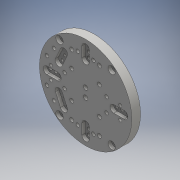
# Autodesk Inventor part: Modular Chassis
Saved by Autodesk Inventor 2016 (Build 200138000, 138)
## iProperties
Created: 2017-03-04
Part Number: Modular Chassis
Material: Generic
Document SubType Name: Modeling
Designer: Billy
Density: 1 g/cm^3
Appearance: Default
Author: Billy
Autodesk Inventor part; units mm, degrees
ref_plane "YZ Plane" through (0, 0, 0) normal (1, 0, 0) x (0, 1, 0)
ref_plane "XZ Plane" through (0, 0, 0) normal (0, 1, 0) x (-1, 0, 0)
ref_plane "XY Plane" through (0, 0, 0) normal (0, 0, 1) x (1, 0, 0)
sketch "Sketch1" plane through (0, 0, 0) normal (0, 1, 0) x (-1, 0, 0)
  circle A0 centre (15.9, 35) radius 2.25
  circle A1 centre (-15.9, 35) radius 2.25
  circle A2 centre (15.9, 16) radius 2.25
  circle A3 centre (-15.9, 16) radius 2.25
  circle A4 centre (0, 0) radius 50.3115
  circle A5 centre (15.9, -35) radius 2.25
  circle A6 centre (-15.9, -35) radius 2.25
  circle A7 centre (15.9, -16) radius 2.25
  circle A8 centre (-15.9, -16) radius 2.25
  circle A9 centre (9, 36.6994) radius 2
  circle A10 centre (-9, 36.6994) radius 2
  circle A11 centre (9, -36.6994) radius 2
  circle A12 centre (-9, -36.6994) radius 2
  circle A13 centre (39.8115, 7.366) radius 1.75
  circle A14 centre (39.8115, -7.366) radius 1.75
  circle A15 centre (-39.8115, 7.366) radius 1.75
  circle A16 centre (-39.8115, -7.366) radius 1.75
  circle A17 centre (27.8558, 21.183) radius 1.5
  circle A18 centre (30.7406, 14.8051) radius 1.5
  circle A19 centre (24.9709, 27.5609) radius 1.5
  circle A20 centre (27.8558, -21.183) radius 1.5
  circle A21 centre (30.7406, -14.8051) radius 1.5
  circle A22 centre (24.9709, -27.5609) radius 1.5
  circle A23 centre (0, 32.3115) radius 2
  circle A24 centre (0, 38.3115) radius 2
  circle A25 centre (0, 44.3115) radius 2
  circle A26 centre (-32.3115, 0) radius 2
  circle A27 centre (-38.3115, 0) radius 2
  circle A28 centre (-44.3115, 0) radius 2
  circle A29 centre (0, -32.3115) radius 2
  circle A30 centre (0, -38.3115) radius 2
  circle A31 centre (0, -44.3115) radius 2
  circle A32 centre (32.3115, 0) radius 2
  circle A33 centre (38.3115, 0) radius 2
  circle A34 centre (44.3115, 0) radius 2
  circle A35 centre (0, 5) radius 2.5
  circle A36 centre (0, -5) radius 2.5
  circle A37 centre (24.1058, 8) radius 2
  circle A38 centre (24.1058, -8) radius 2
  circle A39 centre (-24.1058, 8) radius 2
  circle A40 centre (-24.1058, -8) radius 2
  circle A41 centre (-27.8558, -21.183) radius 2
  circle A42 centre (27.886, -37.3906) radius 2
  line L0 (0, 0) -> (2.5, 0)
  circle A43 centre (27.886, 37.3906) radius 2
  circle A44 centre (44.3115, -14.732) radius 2
  circle A45 centre (44.3115, 14.732) radius 2
  line L1 (-27.8558, -21.183) -> (-36.9207, -29.0268)
  circle A46 centre (-21.8779, -28.0915) radius 2
  circle A47 centre (-33.8336, -14.2745) radius 2
  circle A48 centre (-27.9275, -33.3262) radius 2
  circle A49 centre (-33.9054, -26.4177) radius 2
  circle A50 centre (-39.8833, -19.5092) radius 2
  circle A51 centre (-27.8558, 21.183) radius 2
  circle A52 centre (-21.8779, 28.0915) radius 2
  circle A53 centre (-33.8336, 14.2745) radius 2
  circle A54 centre (-27.9275, 33.3262) radius 2
  circle A55 centre (-33.9054, 26.4177) radius 2
  circle A56 centre (-39.8833, 19.5092) radius 2
  circle A57 centre (36.0988, -26.0613) radius 2
  circle A58 centre (36.0988, 26.0613) radius 2
  point P0 (-36.9207, 29.0268)
  dimension "d47" = 360
  dimension "d64" = 8
  dimension "d69" = 4
  dimension "d70" = 4
  constraints: 59 centre point, 9 symmetric about line, 4 end point, 1 horizontal, 40 other
  measures "d64" distance of A46.centre A48.centre
  measures "d69" diameter of A57
  measures "d70" diameter of A58
extrude "Extrusion1" add sketch "Sketch1" along normal blind 10
sketch "Sketch2" plane through (0, 10, 0) normal (0, 1, 0) x (1, 0, 0)
  circle A0 centre (0, 5) radius 2.5
  circle A1 centre (0, -5) radius 2.5
  circle A2 centre (15.9, 16) radius 2.25
  circle A3 centre (-15.9, 16) radius 2.25
  circle A4 centre (15.9, 35) radius 2.25
  circle A5 centre (-15.9, 35) radius 2.25
  circle A6 centre (15.9, -16) radius 2.25
  circle A7 centre (-15.9, -16) radius 2.25
  circle A8 centre (15.9, -35) radius 2.25
  circle A9 centre (-36.0988, -26.0613) radius 2
  circle A10 centre (-36.0988, 26.0613) radius 2
  circle A11 centre (27.9275, -33.3262) radius 2
  circle A12 centre (39.8833, -19.5092) radius 2
  circle A13 centre (33.8336, -14.2745) radius 2
  circle A14 centre (27.8558, -21.183) radius 2
  circle A15 centre (33.9054, -26.4177) radius 2
  circle A16 centre (21.8779, -28.0915) radius 2
  circle A17 centre (39.8833, 19.5092) radius 2
  circle A18 centre (33.9054, 26.4177) radius 2
  circle A19 centre (27.9275, 33.3262) radius 2
  circle A20 centre (33.8336, 14.2745) radius 2
  circle A21 centre (21.8779, 28.0915) radius 2
  circle A22 centre (-44.3115, -14.732) radius 2
  circle A23 centre (-44.3115, 14.732) radius 2
  circle A24 centre (-27.886, -37.3906) radius 2
  circle A25 centre (-27.886, 37.3906) radius 2
  circle A26 centre (27.8558, 21.183) radius 2
  circle A27 centre (24.1058, 8) radius 2
  circle A28 centre (24.1058, -8) radius 2
  circle A29 centre (-24.1058, 8) radius 2
  circle A30 centre (-24.1058, -8) radius 2
  circle A31 centre (-44.3115, 0) radius 2
  circle A32 centre (-38.3115, 0) radius 2
  circle A33 centre (-32.3115, 0) radius 2
  circle A34 centre (0, 44.3115) radius 2
  circle A35 centre (0, 38.3115) radius 2
  circle A36 centre (0, 32.3115) radius 2
  circle A37 centre (44.3115, 0) radius 2
  circle A38 centre (38.3115, 0) radius 2
  circle A39 centre (32.3115, 0) radius 2
  circle A40 centre (0, -44.3115) radius 2
  circle A41 centre (0, -38.3115) radius 2
  circle A42 centre (0, -32.3115) radius 2
  circle A43 centre (-9, 36.6994) radius 2
  circle A44 centre (9, 36.6994) radius 2
  circle A45 centre (9, -36.6994) radius 2
  circle A46 centre (39.8115, 7.366) radius 1.75
  circle A47 centre (39.8115, -7.366) radius 1.75
  circle A48 centre (-39.8115, 7.366) radius 1.75
  circle A49 centre (-39.8115, -7.366) radius 1.75
  circle A50 centre (-30.7406, 14.8051) radius 1.5
  circle A51 centre (-27.8558, 21.183) radius 1.5
  circle A52 centre (-24.9709, 27.5609) radius 1.5
  circle A53 centre (-24.9709, -27.5609) radius 1.5
  circle A54 centre (-30.7406, -14.8051) radius 1.5
  circle A55 centre (-27.8558, -21.183) radius 1.5
  circle A56 centre (0, 0) radius 50.3115
  circle A57 centre (44.3115, 0) radius 2
  circle A58 centre (38.3115, 0) radius 2
  circle A59 centre (32.3115, 0) radius 2
  circle A60 centre (39.8115, 7.366) radius 1.75
  circle A61 centre (39.8115, -7.366) radius 1.75
  circle A62 centre (-15.9, -16) radius 5
  arc A63 (-14.7043, -30.1451) -> (-17.0957, -39.8549) centre (-15.9, -35) ccw
  arc A64 (-10.1957, -41.5543) -> (-7.8043, -31.8444) centre (-9, -36.6994) ccw
  line L0 (-10.1957, -41.5543) -> (-17.0957, -39.8549)
  circle A65 centre (-15.9, -35) radius 2.25
  circle A66 centre (-9, -36.6994) radius 2
  line L1 (-7.8043, -31.8444) -> (-14.7043, -30.1451)
  line L2 (0, 0) -> (0, -5)
  line L3 (0, 0) -> (-3.6207, 0)
  circle A67 centre (15.9, -16) radius 5
  arc A68 (17.0957, -39.8549) -> (14.7043, -30.1451) centre (15.9, -35) ccw
  arc A69 (7.8043, -31.8444) -> (10.1957, -41.5543) centre (9, -36.6994) ccw
  line L4 (10.1957, -41.5543) -> (17.0957, -39.8549)
  line L5 (7.8043, -31.8444) -> (14.7043, -30.1451)
  circle A70 centre (-15.9, 16) radius 5
  arc A71 (-17.0957, 39.8549) -> (-14.7043, 30.1451) centre (-15.9, 35) ccw
  arc A72 (-7.8043, 31.8444) -> (-10.1957, 41.5543) centre (-9, 36.6994) ccw
  line L6 (-10.1957, 41.5543) -> (-17.0957, 39.8549)
  line L7 (-7.8043, 31.8444) -> (-14.7043, 30.1451)
  arc A73 (14.7043, 30.1451) -> (17.0957, 39.8549) centre (15.9, 35) ccw
  line L8 (7.8043, 31.8444) -> (14.7043, 30.1451)
  arc A74 (10.1957, 41.5543) -> (7.8043, 31.8444) centre (9, 36.6994) ccw
  line L9 (10.1957, 41.5543) -> (17.0957, 39.8549)
  circle A75 centre (15.9, 16) radius 5
  circle A76 centre (-39.8115, 7.366) radius 4.25
  circle A77 centre (-39.8115, -7.366) radius 4.25
  circle A78 centre (39.8115, 7.366) radius 4.25
  circle A79 centre (39.8115, -7.366) radius 4.25
  dimension "d85" = 8.5
  dimension "d86" = 8.5
  dimension "d87" = 8.5
  dimension "d88" = 8.5
  constraints: 141 centre point, 21 symmetric about line, 20 end point, 16 point on circle, 5 coincident, 1 horizontal, 1 vertical, 9 other
  measures "d85" diameter of A76
  measures "d86" diameter of A77
  measures "d87" diameter of A78
  measures "d88" diameter of A79
extrude "Extrusion2" cut sketch "Sketch2" against normal blind 4 contours A62 | L1 A64 L0 A63 | A67 | L4 A69 L5 A68 | A70 | L6 A72 L7 A71 | L8 A74 L9 A73 | A75 | A76 | A77 | A78 | A79
sketch "Sketch3" plane through (0, 0, 0) normal (0, -1, 0) x (1, 0, 0)
  circle A0 centre (0, -5) radius 2.5
  circle A1 centre (0, 5) radius 2.5
  circle A2 centre (15.9, -16) radius 2.25
  circle A3 centre (-15.9, -16) radius 2.25
  circle A4 centre (15.9, -35) radius 2.25
  circle A5 centre (-15.9, -35) radius 2.25
  circle A6 centre (15.9, 16) radius 2.25
  circle A7 centre (-15.9, 16) radius 2.25
  circle A8 centre (15.9, 35) radius 2.25
  circle A9 centre (-15.9, 35) radius 2.25
  circle A10 centre (-36.0988, 26.0613) radius 2
  circle A11 centre (-36.0988, -26.0613) radius 2
  circle A12 centre (27.9275, 33.3262) radius 2
  circle A13 centre (39.8833, 19.5092) radius 2
  circle A14 centre (33.8336, 14.2745) radius 2
  circle A15 centre (27.8558, 21.183) radius 2
  circle A16 centre (33.9054, 26.4177) radius 2
  circle A17 centre (21.8779, 28.0915) radius 2
  circle A18 centre (39.8833, -19.5092) radius 2
  circle A19 centre (33.9054, -26.4177) radius 2
  circle A20 centre (27.9275, -33.3262) radius 2
  circle A21 centre (33.8336, -14.2745) radius 2
  circle A22 centre (21.8779, -28.0915) radius 2
  circle A23 centre (-44.3115, 14.732) radius 2
  circle A24 centre (-44.3115, -14.732) radius 2
  circle A25 centre (-27.886, 37.3906) radius 2
  circle A26 centre (-27.886, -37.3906) radius 2
  circle A27 centre (27.8558, -21.183) radius 2
  circle A28 centre (24.1058, -8) radius 2
  circle A29 centre (24.1058, 8) radius 2
  circle A30 centre (-24.1058, -8) radius 2
  circle A31 centre (-24.1058, 8) radius 2
  circle A32 centre (-44.3115, 0) radius 2
  circle A33 centre (-38.3115, 0) radius 2
  circle A34 centre (-32.3115, 0) radius 2
  circle A35 centre (0, -44.3115) radius 2
  circle A36 centre (0, -38.3115) radius 2
  circle A37 centre (0, -32.3115) radius 2
  circle A38 centre (44.3115, 0) radius 2
  circle A39 centre (38.3115, 0) radius 2
  circle A40 centre (32.3115, 0) radius 2
  circle A41 centre (0, 44.3115) radius 2
  circle A42 centre (0, 38.3115) radius 2
  circle A43 centre (0, 32.3115) radius 2
  circle A44 centre (-9, -36.6994) radius 2
  circle A45 centre (9, -36.6994) radius 2
  circle A46 centre (9, 36.6994) radius 2
  circle A47 centre (-9, 36.6994) radius 2
  circle A48 centre (39.8115, -7.366) radius 1.75
  circle A49 centre (39.8115, 7.366) radius 1.75
  circle A50 centre (-39.8115, -7.366) radius 1.75
  circle A51 centre (-39.8115, 7.366) radius 1.75
  circle A52 centre (-30.7406, -14.8051) radius 1.5
  circle A53 centre (-27.8558, -21.183) radius 1.5
  circle A54 centre (-24.9709, -27.5609) radius 1.5
  circle A55 centre (-24.9709, 27.5609) radius 1.5
  circle A56 centre (-30.7406, 14.8051) radius 1.5
  circle A57 centre (-27.8558, 21.183) radius 1.5
  circle A58 centre (0, 0) radius 50.3115
  arc A59 (-34.6129, 16.5566) -> (-26.8683, 13.0536) centre (-30.7406, 14.8051) ccw
  arc A60 (-21.0986, 25.8094) -> (-28.8432, 29.3124) centre (-24.9709, 27.5609) ccw
  line L0 (-28.8432, 29.3124) -> (-34.6129, 16.5566)
  line L1 (-21.0986, 25.8094) -> (-26.8683, 13.0536)
  line L2 (0, 0) -> (-2, 0)
  arc A61 (-26.8683, -13.0536) -> (-34.6129, -16.5566) centre (-30.7406, -14.8051) ccw
  arc A62 (-28.8432, -29.3124) -> (-21.0986, -25.8094) centre (-24.9709, -27.5609) ccw
  line L3 (-28.8432, -29.3124) -> (-34.6129, -16.5566)
  line L4 (-21.0986, -25.8094) -> (-26.8683, -13.0536)
  arc A63 (-32.3115, -4.25) -> (-32.3115, 4.25) centre (-32.3115, 0) ccw
  line L5 (-44.3115, -4.25) -> (-32.3115, -4.25)
  line L6 (-44.3115, 4.25) -> (-32.3115, 4.25)
  arc A64 (-44.3115, 4.25) -> (-44.3115, -4.25) centre (-44.3115, 0) ccw
  line L7 (0, 0) -> (0, 0.9007)
  arc A65 (32.3115, 4.25) -> (32.3115, -4.25) centre (32.3115, 0) ccw
  line L8 (44.3115, -4.25) -> (32.3115, -4.25)
  line L9 (44.3115, 4.25) -> (32.3115, 4.25)
  arc A66 (44.3115, -4.25) -> (44.3115, 4.25) centre (44.3115, 0) ccw
  arc A67 (-4.25, -44.3115) -> (4.25, -44.3115) centre (0, -44.3115) ccw
  arc A68 (4.25, -32.3115) -> (-4.25, -32.3115) centre (0, -32.3115) ccw
  line L10 (-4.25, -44.3115) -> (-4.25, -32.3115)
  line L11 (4.25, -32.3115) -> (4.25, -44.3115)
  arc A69 (4.25, 44.3115) -> (-4.25, 44.3115) centre (0, 44.3115) ccw
  arc A70 (-4.25, 32.3115) -> (4.25, 32.3115) centre (0, 32.3115) ccw
  line L12 (-4.25, 44.3115) -> (-4.25, 32.3115)
  line L13 (4.25, 32.3115) -> (4.25, 44.3115)
  constraints: 129 centre point, 28 end point, 24 point on circle, 18 symmetric about line, 6 coincident, 3 tangent, 2 horizontal, 1 vertical, 6 other
extrude "Extrusion3" cut sketch "Sketch3" against normal blind 4 contours L0 A60 L1 A59 | L4 A62 L3 A61 | L5 A64 L6 A63 | L9 A66 L8 A65 | L10 A68 L11 A67 | L13 A70 L12 A69
sketch "Sketch4" plane through (0, 10, 0) normal (0, 1, 0) x (1, 0, 0)
  circle A0 centre (-27.886, -37.3906) radius 2 projected
  circle A1 centre (-27.886, 37.3906) radius 2 projected
  point P0 (0, 0)
extrude "Extrusion4" add sketch "Sketch4" against normal blind 10
sketch "Sketch5" plane through (0, 10, 0) normal (0, 1, 0) x (1, 0, 0)
  line L0 (0, 0) -> (-30, 0)
  line L1 (-30, 37.5) -> (0, 37.5)
  line L2 (0, 37.5) -> (0, 0)
  line L3 (30, -37.5) -> (-30, -37.5)
  circle A0 centre (-30, -37.5) radius 2
  circle A1 centre (-30, 37.5) radius 2
  circle A2 centre (30, -37.5) radius 2
  circle A3 centre (30, 37.5) radius 2
  dimension "d104" = 30
  dimension "d105" = 37.5
  dimension "d106" = 60
  dimension "d108" = 4
  dimension "d109" = 4
  dimension "d110" = 4
  dimension "d111" = 4
  constraints: 8 end point, 4 centre point, 3 coincident, 1 horizontal, 1 parallel
  measures "d104" distance of L1.start L1.end
  measures "d105" distance of L0.end L1.start
  measures "d106" distance of L3.start L3.end
  measures "d108" diameter of A0
  measures "d109" diameter of A1
  measures "d110" diameter of A2
  measures "d111" diameter of A3
extrude "Extrusion5" cut sketch "Sketch5" against normal blind 10
sketch "Sketch6" plane through (0, 10, 0) normal (0, 1, 0) x (1, 0, 0)
  circle A0 centre (0, 0) radius 50.3115 projected
  circle A1 centre (27.8558, 21.183) radius 2 projected
  circle A2 centre (30, -37.5) radius 2 projected
  circle A3 centre (-30, -37.5) radius 2 projected
  circle A4 centre (-30, 37.5) radius 2 projected
  circle A5 centre (30, 37.5) radius 2 projected
  line L0 (-17.0957, 39.8549) -> (-10.1957, 41.5543) projected
  arc A6 (-7.8043, 31.8444) -> (-10.1957, 41.5543) centre (-9, 36.6994) ccw projected
  line L1 (-7.8043, 31.8444) -> (-14.7043, 30.1451) projected
  arc A7 (-17.0957, 39.8549) -> (-14.7043, 30.1451) centre (-15.9, 35) ccw projected
  line L2 (-14.7043, -30.1451) -> (-7.8043, -31.8444) projected
  arc A8 (-10.1957, -41.5543) -> (-7.8043, -31.8444) centre (-9, -36.6994) ccw projected
  line L3 (-10.1957, -41.5543) -> (-17.0957, -39.8549) projected
  arc A9 (-14.7043, -30.1451) -> (-17.0957, -39.8549) centre (-15.9, -35) ccw projected
  circle A10 centre (-15.9, 16) radius 5 projected
  circle A11 centre (-15.9, -16) radius 5 projected
  circle A12 centre (39.8115, 7.366) radius 4.25 projected
  circle A13 centre (-39.8115, 7.366) radius 4.25 projected
  circle A14 centre (-39.8115, -7.366) radius 4.25 projected
  circle A15 centre (39.8115, -7.366) radius 4.25 projected
  circle A16 centre (15.9, -16) radius 5 projected
  circle A17 centre (15.9, 16) radius 5 projected
  arc A18 (7.8043, -31.8444) -> (10.1957, -41.5543) centre (9, -36.6994) ccw projected
  line L4 (7.8043, -31.8444) -> (14.7043, -30.1451) projected
  arc A19 (17.0957, -39.8549) -> (14.7043, -30.1451) centre (15.9, -35) ccw projected
  line L5 (17.0957, -39.8549) -> (10.1957, -41.5543) projected
  arc A20 (14.7043, 30.1451) -> (17.0957, 39.8549) centre (15.9, 35) ccw projected
  line L6 (14.7043, 30.1451) -> (7.8043, 31.8444) projected
  arc A21 (10.1957, 41.5543) -> (7.8043, 31.8444) centre (9, 36.6994) ccw projected
  line L7 (10.1957, 41.5543) -> (17.0957, 39.8549) projected
  circle A22 centre (0, 5) radius 2.5 projected
  circle A23 centre (0, -5) radius 2.5 projected
  circle A24 centre (-36.0988, -26.0613) radius 2 projected
  circle A25 centre (-36.0988, 26.0613) radius 2 projected
  circle A26 centre (27.9275, -33.3262) radius 2 projected
  circle A27 centre (39.8833, -19.5092) radius 2 projected
  circle A28 centre (33.8336, -14.2745) radius 2 projected
  circle A29 centre (27.8558, -21.183) radius 2 projected
  circle A30 centre (33.9054, -26.4177) radius 2 projected
  circle A31 centre (21.8779, -28.0915) radius 2 projected
  circle A32 centre (39.8833, 19.5092) radius 2 projected
  circle A33 centre (33.9054, 26.4177) radius 2 projected
  circle A34 centre (27.9275, 33.3262) radius 2 projected
  circle A35 centre (33.8336, 14.2745) radius 2 projected
  circle A36 centre (21.8779, 28.0915) radius 2 projected
  circle A37 centre (-44.3115, -14.732) radius 2 projected
  circle A38 centre (-44.3115, 14.732) radius 2 projected
  circle A39 centre (27.8558, 21.183) radius 2 projected
  circle A40 centre (24.1058, 8) radius 2 projected
  circle A41 centre (24.1058, -8) radius 2 projected
  circle A42 centre (-24.1058, 8) radius 2 projected
  circle A43 centre (-24.1058, -8) radius 2 projected
  circle A44 centre (-44.3115, 0) radius 2 projected
  circle A45 centre (-38.3115, 0) radius 2 projected
  circle A46 centre (-32.3115, 0) radius 2 projected
  circle A47 centre (0, 44.3115) radius 2 projected
  circle A48 centre (0, 38.3115) radius 2 projected
  circle A49 centre (0, 32.3115) radius 2 projected
  circle A50 centre (44.3115, 0) radius 2 projected
  circle A51 centre (38.3115, 0) radius 2 projected
  circle A52 centre (32.3115, 0) radius 2 projected
  circle A53 centre (0, -44.3115) radius 2 projected
  circle A54 centre (0, -38.3115) radius 2 projected
  circle A55 centre (0, -32.3115) radius 2 projected
  circle A56 centre (-30.7406, 14.8051) radius 1.5 projected
  circle A57 centre (-27.8558, 21.183) radius 1.5 projected
  circle A58 centre (-24.9709, 27.5609) radius 1.5 projected
  circle A59 centre (-24.9709, -27.5609) radius 1.5 projected
  circle A60 centre (-30.7406, -14.8051) radius 1.5 projected
  circle A61 centre (-27.8558, -21.183) radius 1.5 projected
  circle A62 centre (0, 0) radius 50.3115 projected
  circle A63 centre (0, 0) radius 53
  dimension "d115" = 106
  constraints: 1 centre point, 1 coincident
  measures "d115" diameter of A63
extrude "Extrusion6" add sketch "Sketch6" against normal blind 10 contours A1 | A26 | A27 | A28 | A29 | A30 | A31 | A32 | A33 | A34 | A35 | A36 | A63
sketch "Sketch8" plane through (0, 0, 0) normal (0, -1, 0) x (1, 0, 0)
  circle A0 centre (30, -37.5) radius 2 projected
  circle A1 centre (30, -37.5) radius 4.25
  circle A2 centre (30, 37.5) radius 2 projected
  circle A3 centre (30, 37.5) radius 4.25
  circle A4 centre (-30, 37.5) radius 2 projected
  circle A5 centre (-30, 37.5) radius 4.25
  circle A6 centre (-30, -37.5) radius 2 projected
  circle A7 centre (-30, -37.5) radius 4.25
  point P0 (0, 0)
  dimension "d118" = 8.5
  dimension "d119" = 8.5
  dimension "d120" = 8.5
  dimension "d121" = 8.5
  constraints: 4 centre point, 4 coincident
  measures "d118" diameter of A1
  measures "d119" diameter of A3
  measures "d120" diameter of A5
  measures "d121" diameter of A7
extrude "Extrusion7" cut sketch "Sketch8" against normal blind 4
body "Solid1"
